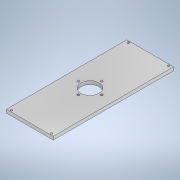
# Autodesk Inventor part: FWheel Side2
Saved by Autodesk Inventor 2020.2 (Build 242310000, 310)
## iProperties
Created: 2020-03-28
Part Number: FWheel Side2
Material: Aluminum 6061-AHC
Document SubType Name: Modeling
Designer: introbot
Density: 2.7 g/cm^3
Appearance: Aluminum - Dark
Mass: 167.073 g
Surface Area: 278.91 cm^2
Volume: 61.8787 cm^3
Author: introbot
Autodesk Inventor part; units mm, degrees
ref_plane "YZ Plane" through (0, 0, 0) normal (1, 0, 0) x (0, 1, 0)
ref_plane "XZ Plane" through (0, 0, 0) normal (0, 1, 0) x (-1, 0, 0)
ref_plane "XY Plane" through (0, 0, 0) normal (0, 0, 1) x (1, 0, 0)
sketch "Sketch1" plane through (0, 0, 0) normal (0, 1, 0) x (-1, 0, 0)
  line L0 (35, 90) -> (-35, 90)
  line L1 (-35, 90) -> (-35, -90)
  line L2 (-35, -90) -> (35, -90)
  line L3 (35, -90) -> (35, 90)
  line L4 (69.6704, 0) -> (-52.4451, 0) projected
  line L5 (0, -129.3465) -> (0, 126.5577) projected
  point P0 (0, 0)
  dimension "d0" = 180
  dimension "d1" = 70
  constraints: 8 end point, 2 parallel, 1 horizontal, 1 perpendicular, 2 other
  measures "d0" distance of L2.end L0.start
  measures "d1" distance of L0.start L0.end
extrude "Extrusion1" add sketch "Sketch1" along normal blind 5
sketch "Sketch2" plane through (0, 5, 0) normal (0, 1, 0) x (1, 0, 0)
  line L0 (-35, 90) -> (-35, -90) projected
  line L1 (35, -90) -> (35, 90) projected
  line L2 (-35, -90) -> (35, -90) projected
  line L3 (-35, -90) -> (35, -90) projected
  line L4 (35, -90) -> (35, 90) projected
  line L5 (35, 90) -> (-35, 90) projected
  line L6 (-35, 90) -> (-35, -90) projected
  line L7 (-49, 0) -> (49, 0) projected
  line L8 (0, 126) -> (0, -126) projected
  point P0 (0, 0)
  point P1 (-30, -87.5)
  point P2 (-30, 87.5)
  point P3 (30, -87.5)
  point P4 (30, 87.5)
  dimension "d4" = 5
  dimension "d5" = 2.5
  constraints: 3 symmetric about line
  measures "d4" distance from line of L0 point (-30, -87.5)
  measures "d5" distance from line of point (-30, -87.5) L2
hole "Hole1" at (-30, 5, -87.5) at (30, 5, 87.5) at (30, 5, -87.5) at (-30, 5, 87.5) direction (0, -1, 0) diameter 3 depth 8.8 tip angle 118
sketch "Sketch3" plane through (0, 5, 0) normal (0, 1, 0) x (1, 0, 0)
  point P0 (0, 0)
hole "Hole2" at (0, 5, 0) direction (0, -1, 0) diameter 27 depth 14.2 tip angle 118
sketch "Sketch5" plane through (0, 5, 0) normal (0, 1, 0) x (1, 0, 0)
  point P0 (0, 0)
sketch "스케치7" plane through (0, 0, 0) normal (0, -1, 0) x (1, 0, 0)
  circle A0 centre (0, 0) radius 17.5
  line L0 (-49, 0) -> (49, 0) projected
  line L1 (0, -126) -> (0, 126) projected
  point P0 (17.5, 0)
  point P1 (0, 17.5)
  point P2 (-17.5, 0)
  point P3 (0, -17.5)
  dimension "d46" = 35
  constraints: 4 point on line, 2 point on circle, 1 centre point, 1 coincident
  measures "d46" diameter of A0
hole "구멍5" at (0, 0, -17.5) at (-17.5, 0, 0) at (0, 0, 17.5) at (17.5, 0, 0) direction (0, 1, 0) diameter 3.242 depth 14.2 tip angle 118
body "Solid1"
